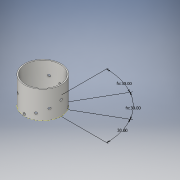
# Autodesk Inventor part: vexFrisbeeHopper
Saved by Autodesk Inventor 2016 (Build 200138000, 138)
## iProperties
Created: 2015-07-20
Part Number: vexFrisbeeHopper
Material: PC/ABS Plastic
Document SubType Name: Modeling
Designer: steele
Density: 0.357273 g/cm^3
Appearance: Smooth - White
Mass: 146.454 g
Surface Area: 2639.82 cm^2
Volume: 409.921 cm^3
Author: steele
Autodesk Inventor part; units mm, degrees
ref_plane "YZ Plane" through (0, 0, 0) normal (1, 0, 0) x (0, 1, 0)
sketch "Sketch1" plane through (0, 0, 0) normal (0, 1, 0) x (-1, 0, 0)
  circle A0 centre (0, 0) radius 49.741667
  circle A1 centre (0, 0) radius 52.916667
  circle A2 centre (0, 0) radius 419.1 construction
  dimension "interiorDiam" = 99.48333
  dimension "exteriorDiam" = 105.83333
  dimension "frisbeeDiam" = 838.2
  constraints: 3 centre point, 3 coincident
  measures "interiorDiam" diameter of A0
  measures "exteriorDiam" diameter of A1
  measures "frisbeeDiam" diameter of A2
extrude "Extrusion1" add sketch "Sketch1" along normal blind 78.74
ref_plane "Work Plane1" through (0, 0, 52.916667) normal (0, 0, 1) x (1, 0, 0)
sketch "Sketch2" plane through (0, 0, 52.916667) normal (0, 0, 1) x (1, 0, 0)
  circle A0 centre (0, 5.926667) radius 3.429
  point P0 (0, 0)
  dimension "xpostHoleDiam" = 6.858
  dimension "firstHoleHeight" = 5.92667
  constraints: 1 centre point
  measures "xpostHoleDiam" diameter of A0
  measures "firstHoleHeight" distance of A0.centre point (0, 0)
extrude "Extrusion2" cut sketch "Sketch2" against normal up to next
pattern_circular "Circular Pattern1" count 3 over 360 about axis through (0, -10, 0) along (0, 1, 0) of "Extrusion2"
sketch "Sketch for Plane" plane through (0, 0, 0) normal (0, 1, 0) x (-1, 0, 0)
  circle A0 centre (0, 0) radius 52.916667 construction
  line L0 (0, 0) -> (-52.916667, 0) construction
  line L1 (0, 0) -> (-45.827178, -26.458333) construction
  line L2 (0, 0) -> (-26.458333, -45.827178) construction
  line L3 (0, 0) -> (0, -52.916667) construction
  dimension "secondHolePlaneAngle" = 30
  dimension "thirdHolePlaneAngle" = 30
  dimension "fourthHolePlaneAngle" = 30
  constraints: 8 end point, 4 point on circle, 1 horizontal
  measures "secondHolePlaneAngle" angle of L1 L0
  measures "thirdHolePlaneAngle" angle of L2 L1
  measures "fourthHolePlaneAngle" angle of L3 L2
ref_plane "Work Plane3" through (26.458333, 0, 45.827178) normal (0.5, 0, 0.8660254) x (0.8660254, 0, -0.5)
ref_plane "Work Plane2" through (0, 0, 0) normal (0.5, 0, 0.8660254) x (0.8660254, 0, -0.5)
sketch "Sketch5" plane through (26.458333, 0, 45.827178) normal (0.5, 0, 0.8660254) x (0.8660254, 0, -0.5)
  circle A0 centre (0, 17.78) radius 3.429
  line L0 (-52.916667, 0) -> (52.916667, 0)
  point P0 (0, 0)
  dimension "secondHoleHeight" = 17.78
  dimension "secondPostHoleDiam" = 6.858
  constraints: 1 centre point
  measures "secondHoleHeight" distance from line of L0 A0.centre
  measures "secondPostHoleDiam" diameter of A0
extrude "Extrusion3" cut sketch "Sketch5" against normal up to next
pattern_circular "Circular Pattern2" count 3 over 360 about axis through (0, -10, 0) along (0, 1, 0) of "Extrusion3"
ref_plane "Work Plane5" through (45.827178, 0, 26.458333) normal (0.8660254, 0, 0.5) x (0.5, 0, -0.8660254)
ref_plane "Work Plane4" through (0, 0, 0) normal (0.8660254, 0, 0.5) x (0.5, 0, -0.8660254)
sketch "Sketch7" plane through (45.827178, 0, 26.458333) normal (0.8660254, 0, 0.5) x (0.5, 0, -0.8660254)
  circle A0 centre (0, 29.633333) radius 3.429
  point P0 (0, 0)
  dimension "thirdPostHoleDiam" = 6.858
  dimension "thirdHoleHeight" = 29.63333
  constraints: 1 centre point
  measures "thirdPostHoleDiam" diameter of A0
  measures "thirdHoleHeight" distance of point (0, 0) A0.centre
extrude "Extrusion4" cut sketch "Sketch7" against normal up to next
pattern_circular "Circular Pattern3" count 3 over 360 about axis through (0, -10, 0) along (0, 1, 0) of "Extrusion4"
ref_plane "Work Plane7" through (52.916667, 0, 0) normal (1, 0, 0) x (0, 0, -1)
ref_plane "Work Plane6" through (0, 0, 0) normal (1, 0, 0) x (0, 0, -1)
sketch "Sketch8" plane through (52.916667, 0, 0) normal (1, 0, 0) x (0, 0, -1)
  circle A0 centre (0, 41.486667) radius 3.429
  point P0 (0, 0)
  dimension "fourthPostHoleDiam" = 6.858
  dimension "fourthHoleHeight" = 41.48667
  constraints: 1 centre point
  measures "fourthPostHoleDiam" diameter of A0
  measures "fourthHoleHeight" distance of point (0, 0) A0.centre
extrude "Extrusion5" cut sketch "Sketch8" against normal up to next
pattern_circular "Circular Pattern4" count 3 over 360 about axis through (0, -10, 0) along (0, 1, 0) of "Extrusion5"
equation "\"xpostHoleDiam\" = postHoleDiam"
equation "\"firstHoleHeight\" = 0.5 * vexFrisbeeHeight"
equation "\"thirdHolePlaneAngle\" = secondHolePlaneAngle"
equation "\"fourthHolePlaneAngle\" = secondHolePlaneAngle"
equation "\"secondHoleHeight\" = firstHoleHeight + vexFrisbeeHeight"
equation "\"secondPostHoleDiam\" = xpostHoleDiam"
equation "\"thirdPostHoleDiam\" = xpostHoleDiam"
equation "\"thirdHoleHeight\" = secondHoleHeight + vexFrisbeeHeight"
equation "\"fourthPostHoleDiam\" = xpostHoleDiam"
equation "\"fourthHoleHeight\" = thirdHoleHeight + vexFrisbeeHeight"
equation "\"d15\" = outsideRadius"
equation "\"outsideRadius\" = 0.5 * exteriorDiam"
equation "\"d35\" = outsideRadius"
equation "\"regulationFrisbeeDiam\" = 279.4"
equation "\"vexFrisbeeDiam\" = 0.333333 * regulationFrisbeeDiam"
equation "\"regulationFrisbeeHeight\" = 35.56"
equation "\"vexFrisbeeHeight\" = 0.333333 * regulationFrisbeeHeight"
equation "\"postHoleDiam\" = 6.858"
body "Solid1"
